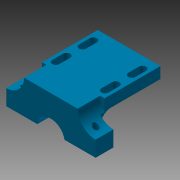
# Autodesk Inventor part: Part15
Saved by Autodesk Inventor 2015 (Build 190159000, 159)
## iProperties
Created: 2015-07-08
Part Number: Part15
Material: ABS Plastic
Document SubType Name: Modeling
Designer: eefred
Density: 1.06 g/cm^3
Appearance: Smooth - Yellow
Author: eefred
Autodesk Inventor part; units mm, degrees
ref_plane "YZ Plane" through (0, 0, 0) normal (1, 0, 0) x (0, 1, 0)
ref_plane "XZ Plane" through (0, 0, 0) normal (0, 1, 0) x (-1, 0, 0)
ref_plane "XY Plane" through (0, 0, 0) normal (0, 0, 1) x (1, 0, 0)
sketch "Sketch1" plane through (0, 0, 0) normal (0, 0, 1) x (1, 0, 0)
  line L0 (-14, 8) -> (14, 8)
  line L1 (14, 8) -> (14, 35)
  line L2 (14, 35) -> (-14, 35)
  line L3 (-14, 35) -> (-14, 8)
  point P0 (0, 0)
  point P1 (0, 8)
  dimension "d0" = 27
  dimension "d1" = 28
  dimension "d2" = 8
  constraints: 8 end point, 2 parallel, 1 horizontal, 1 midpoint, 1 perpendicular, 1 vertical alignment
  measures "d0" distance of L1.end L0.end
  measures "d1" distance of L1.end L2.end
  measures "d2" distance from line of point (0, 0) L0
extrude "Extrusion1" add sketch "Sketch1" along normal blind 5
sketch "Sketch2" plane through (0, 0, 5) normal (0, 0, 1) x (1, 0, 0)
  line L0 (-20, 0) -> (20, 0)
  line L1 (20, 0) -> (20, 8)
  line L2 (20, 8) -> (-20, 8)
  line L3 (-20, 8) -> (-20, 0)
  point P0 (0, 0)
  point P1 (0, 0)
  dimension "d7" = 40
  dimension "d8" = 8
  constraints: 8 end point, 2 parallel, 1 coincident, 1 horizontal, 1 horizontal alignment, 1 midpoint, 1 perpendicular
  measures "d7" distance of L2.end L1.end
  measures "d8" distance of L1.end L0.end
extrude "Extrusion2" add sketch "Sketch2" against normal blind 15
fillet "Fillet1" radius 5 1 edges at (0, 8, 0)
sketch "Sketch3" plane through (0, 0, 5) normal (0, 0, 1) x (1, 0, 0)
  line L0 (-11, 31.6) -> (-11, 31.6)
  line L1 (-9.4, 30) -> (-9.4, 25.2)
  line L2 (-11, 23.6) -> (-11, 23.6)
  line L3 (-12.6, 25.2) -> (-12.6, 30)
  arc A0 (-12.6, 25.2) -> (-11, 23.6) centre (-11, 25.2) ccw
  arc A1 (-11, 23.6) -> (-9.4, 25.2) centre (-11, 25.2) ccw
  arc A2 (-9.4, 30) -> (-11, 31.6) centre (-11, 30) ccw
  arc A3 (-11, 31.6) -> (-12.6, 30) centre (-11, 30) ccw
  line L4 (-14, 35) -> (-14, 8) projected
  line L5 (14, 35) -> (-14, 35) projected
  point P0 (0, 0)
  point P1 (-9.4, 23.6)
  point P2 (-9.4, 31.6)
  point P3 (-12.6, 23.6)
  dimension "d12" = 3.2
  dimension "d13" = 8
  dimension "d14" = 1.6
  dimension "d15" = 3
  dimension "d16" = 5
  constraints: 8 end point, 8 point on circle, 8 tangent, 6 point on line, 4 centre point, 3 equal radius, 2 parallel, 1 horizontal, 1 perpendicular
  measures "d12" distance of point (-9.4, 23.6) point (-12.6, 23.6)
  measures "d13" distance of point (-9.4, 31.6) point (-9.4, 23.6)
  measures "d14" radius of A0
  measures "d15" distance from line of L4 A2.centre
  measures "d16" distance from line of L5 A2.centre
extrude "Extrusion3" cut sketch "Sketch3" against normal blind 10
pattern_linear "Rectangular Pattern1" count 2 spacing 12 along (0, -1, 0) count 2 spacing 22 along (1, 0, 0) of "Extrusion3"
sketch "Sketch4" plane through (14, 8, 5) normal (0, 1, 0) x (1, 0, 0)
  arc A0 (-20.15, 16) -> (-7.85, 16) centre (-14, 16) ccw
  line L0 (-7.85, 16) -> (-20.15, 16)
  line L1 (-34, 15) -> (6, 15) projected
  point P0 (-14, 5)
  point P1 (-14, 15)
  dimension "d25" = 6.15
  dimension "d26" = 1
  constraints: 2 end point, 2 midpoint, 2 point on circle, 1 centre point, 1 horizontal, 1 horizontal alignment, 1 vertical alignment
  measures "d25" radius of A0
  measures "d26" distance of A0.centre point (-14, 15)
extrude "Extrusion4" cut sketch "Sketch4" along normal through all both and the other way through all
sketch "Sketch5" plane through (14, 8, 5) normal (0, 1, 0) x (1, 0, 0)
  arc A0 (-12.65, 10) -> (-7.9318, 15) centre (-14, 16) ccw construction
  arc A1 (-21.65, 16) -> (-6.35, 16) centre (-14, 16) ccw
  line L0 (-21.65, 16) -> (-6.35, 16)
  point P0 (-14, 5)
  dimension "d29" = 7.65
  constraints: 2 end point, 2 horizontal alignment, 2 point on circle, 1 centre point, 1 coincident
  measures "d29" radius of A1
extrude "Extrusion5" cut sketch "Sketch5" against normal blind 3 and the other way blind 1
sketch "Sketch6" plane through (-14, 35, 0) normal (0, 1, 0) x (1, 0, 0)
  arc A0 (7.9318, 10) -> (20.0682, 10) centre (14, 11) ccw construction
  arc A1 (1.25, 11) -> (26.75, 11) centre (14, 11) ccw
  line L0 (26.75, 11) -> (1.25, 11)
  point P0 (14, 0)
  dimension "d34" = 12.75
  constraints: 2 end point, 2 horizontal alignment, 2 point on circle, 1 centre point, 1 coincident
  measures "d34" radius of A1
extrude "Extrusion6" cut sketch "Sketch6" against normal blind 23
sketch "Sketch7" plane through (0, 0, -10) normal (0, 0, -1) x (-1, 0, 0)
  circle A0 centre (-16, 4) radius 1.3
  circle A1 centre (16, 4) radius 1.3
  line L0 (-20, 0) -> (-6.0682, 0) projected
  line L1 (-20, 8) -> (-20, 0) projected
  line L2 (20, 0) -> (20, 8) projected
  point P0 (0, 0)
  dimension "d37" = 2.6
  dimension "d38" = 4
  dimension "d39" = 4
  dimension "d40" = 4
  constraints: 2 centre point, 1 equal radius, 1 horizontal alignment
  measures "d37" diameter of A0
  measures "d38" distance from line of L0 A0.centre
  measures "d39" distance from line of A0.centre L1
  measures "d40" distance from line of L2 A1.centre
extrude "Extrusion7" cut sketch "Sketch7" against normal through all
sketch "Sketch8" plane through (-20, 0, 5) normal (0, -1, 0) x (1, 0, 0)
  circle A0 centre (40, 0) radius 8
  circle A1 centre (0, 0) radius 8
  point P0 (20, -5)
  dimension "d43" = 16
  dimension "d44" = 16
  constraints: 2 centre point, 1 coincident
  measures "d43" diameter of A0
  measures "d44" diameter of A1
extrude "Extrusion8" cut sketch "Sketch8" against normal blind 10
equation "\"d40\" = d39"
body "Solid1"
